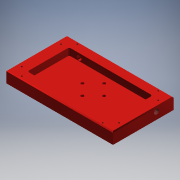
# Autodesk Inventor part: UNLHEP-14-01-P-004_ChuckForGantry
Saved by Autodesk Inventor 2019.4 (Build 234330000, 330)
## iProperties
Created: 2014-01-09
Part Number: UNLHEP-14-01-P-004_ChuckForGantry
Material: Aluminum, Anodized Red
Document SubType Name: Modeling
Designer: Frank Meier
Density: 2.7 g/cm^3
Project: UNL Pixel Phase I
Mass: 2699.72 g
Surface Area: 1115.91 cm^2
Volume: 999.896 cm^3
Appearance: Anodized - Red
Author: Frank Meier
Revision Number: 00
Autodesk Inventor part; units mm, degrees
ref_plane "YZ Plane" through (0, 0, 0) normal (1, 0, 0) x (0, 1, 0)
ref_plane "XZ Plane" through (0, 0, 0) normal (0, 1, 0) x (-1, 0, 0)
ref_plane "XY Plane" through (0, 0, 0) normal (0, 0, 1) x (1, 0, 0)
sketch "Skizze1" plane through (0, 0, 0) normal (0, 0, 1) x (1, 0, 0)
  line L0 (-123, -70) -> (123, -70)
  line L1 (123, -70) -> (123, 70)
  line L2 (123, 70) -> (-123, 70)
  line L3 (-123, 70) -> (-123, -70)
  line L4 (-123, -70) -> (123, 70) construction
  line L5 (123, -70) -> (-123, 70) construction
  point P0 (0, 0)
  dimension "d0" = 246
  dimension "d2" = 140
  constraints: 12 end point, 2 midpoint, 2 parallel, 1 horizontal, 1 perpendicular
  measures "d0" distance of L1.end L2.end
  measures "d2" distance of L0.end L1.end
extrude "Extrusion1" add sketch "Skizze1" along normal blind 26
sketch "Skizze2" plane through (0, 0, 26) normal (0, 0, 1) x (1, 0, 0)
  line L0 (-96, -48) -> (96, -48)
  line L1 (96, -48) -> (96, 48)
  line L2 (96, 48) -> (-96, 48)
  line L3 (-96, 48) -> (-96, -48)
  line L4 (-96, -48) -> (96, 48) construction
  line L5 (96, -48) -> (-96, 48) construction
  line L6 (-123, -70) -> (123, -70) projected
  line L7 (123, -70) -> (123, 70) projected
  line L8 (123, 70) -> (-123, 70) projected
  line L9 (-123, 70) -> (-123, -70) projected
  circle A0 centre (-115, 40) radius 2
  circle A1 centre (-93, 62) radius 2
  circle A2 centre (93, 62) radius 2
  circle A3 centre (115, 40) radius 2
  circle A4 centre (115, -40) radius 2
  circle A5 centre (93, -62) radius 2
  circle A6 centre (-93, -62) radius 2
  circle A7 centre (-115, -40) radius 2
  point P0 (0, 0)
  dimension "d5" = 192
  dimension "d7" = 96
  dimension "d14" = 8
  dimension "d15" = 30
  dimension "d16" = 30
  dimension "d17" = 8
  dimension "d18" = 8
  dimension "d19" = 30
  dimension "d20" = 8
  dimension "d21" = 30
  dimension "d22" = 30
  dimension "d23" = 8
  dimension "d24" = 8
  dimension "d25" = 30
  dimension "d26" = 8
  dimension "d27" = 30
  dimension "d28" = 30
  dimension "d29" = 8
  dimension "d30" = 4
  dimension "d31" = 4
  dimension "d32" = 4
  dimension "d33" = 4
  dimension "d34" = 4
  dimension "d35" = 4
  dimension "d36" = 4
  dimension "d37" = 4
  constraints: 12 end point, 8 centre point, 8 coincident, 2 midpoint, 2 parallel, 1 horizontal, 1 perpendicular
  measures "d5" distance of L1.end L2.end
  measures "d7" distance of L0.end L1.end
  measures "d14" distance from line of L9 point (-115, 40)
  measures "d15" distance from line of L8 point (-115, 40)
  measures "d16" distance from line of L9 point (-93, 62)
  measures "d17" distance from line of L8 point (-93, 62)
  measures "d18" distance from line of L8 point (93, 62)
  measures "d19" distance from line of L7 point (93, 62)
  measures "d20" distance from line of L7 point (115, 40)
  measures "d21" distance from line of L8 point (115, 40)
  measures "d22" distance from line of L6 point (115, -40)
  measures "d23" distance from line of L7 point (115, -40)
  measures "d24" distance from line of L6 point (93, -62)
  measures "d25" distance from line of L7 point (93, -62)
  measures "d26" distance from line of L6 point (-93, -62)
  measures "d27" distance from line of L9 point (-93, -62)
  measures "d28" distance from line of L6 point (-115, -40)
  measures "d29" distance from line of L9 point (-115, -40)
  measures "d30" diameter of A0
  measures "d31" diameter of A1
  measures "d32" diameter of A2
  measures "d33" diameter of A3
  measures "d34" diameter of A4
  measures "d35" diameter of A5
  measures "d36" diameter of A6
  measures "d37" diameter of A7
extrude "Extrusion2" cut sketch "Skizze2" against normal blind 16 contours L3 L2 L1 L0
fillet "Rundung1" radius 4 4 edges at (-96, 48, 18) (96, 48, 18) (96, -48, 18) (-96, -48, 18)
chamfer "Fase1" distance 2 angle 45 4 edges at (0, -70, 26) (-123, 0, 26) (0, 70, 26) (123, 0, 26)
sketch "Skizze4" plane through (0, 0, 26) normal (0, 0, 1) x (1, 0, 0)
  line L0 (123, 70) -> (-123, 70) projected
  line L1 (123, -70) -> (123, 70) projected
  line L2 (-123, 70) -> (-123, -70) projected
  line L3 (-123, -70) -> (123, -70) projected
  point P0 (-112, 45)
  point P1 (-112, -45)
  point P2 (-93, -64)
  point P3 (-93, 64)
  point P4 (93, 64)
  point P5 (112, 45)
  point P6 (112, -45)
  point P7 (93, -64)
  dimension "d153" = 25
  dimension "d154" = 25
  dimension "d155" = 11
  dimension "d156" = 6
  dimension "d157" = 30
  dimension "d158" = 11
  dimension "d159" = 6
  dimension "d160" = 30
  dimension "d161" = 30
  dimension "d162" = 6
  dimension "d163" = 11
  dimension "d164" = 25
  dimension "d165" = 11
  dimension "d166" = 25
  dimension "d167" = 6
  dimension "d168" = 30
  measures "d153" distance from line of L0 point (-112, 45)
  measures "d154" distance from line of L3 point (-112, -45)
  measures "d155" distance from line of L2 point (-112, -45)
  measures "d156" distance from line of L3 point (-93, -64)
  measures "d157" distance from line of L2 point (-93, -64)
  measures "d158" distance from line of L2 point (-112, 45)
  measures "d159" distance from line of L0 point (-93, 64)
  measures "d160" distance from line of L2 point (-93, 64)
  measures "d161" distance from line of L1 point (93, 64)
  measures "d162" distance from line of L0 point (93, 64)
  measures "d163" distance from line of L1 point (112, 45)
  measures "d164" distance from line of L0 point (112, 45)
  measures "d165" distance from line of L1 point (112, -45)
  measures "d166" distance from line of L3 point (112, -45)
  measures "d167" distance from line of L3 point (93, -64)
  measures "d168" distance from line of L1 point (93, -64)
sketch "Sketch10" plane through (123, -70, 0) normal (1, 0, 0) x (0, 0, -1)
  line L0 (-26, 138) -> (-26, 2) projected
  line L1 (0, 0) -> (-24, 0) projected
  line L2 (0, 0) -> (0, 140) projected
  point P0 (-16, 100)
  dimension "d93" = 100
  dimension "d215" = 16
  measures "d93" distance from line of L1 point (-16, 100)
  measures "d215" distance from line of L2 point (-16, 100)
hole "Bohrung3" at (123, 30, 16) direction (-1, 0, 0) diameter 10.719 depth 27 tip angle 118 taper from width 11.358 to width 10.732 over 10.02 thread size "1/4" designation "1/4 - 18 NPT" standard "NPT"
hole "Bohrung7" at (-93, 64, 26) at (-112, 45, 26) at (-112, -45, 26) at (-93, -64, 26) at (93, 64, 26) at (112, 45, 26) at (112, -45, 26) at (93, -64, 26) direction (0, 0, -1) diameter 3.242 depth 20 tip angle 118 thread size "M4x0.7" class "6H" standard "ISO Metric profile"
sketch "Sketch11" plane through (-123, 70, 0) normal (0, 1, 0) x (1, 0, 0)
  line L0 (246, 0) -> (0, 0) projected
  line L1 (0, 0) -> (0, -24) projected
  point P0 (123, 0)
  point P1 (50, -16)
  dimension "d182" = 16
  dimension "d183" = 50
  measures "d182" distance from line of L0 point (50, -16)
  measures "d183" distance from line of L1 point (50, -16)
hole "Hole8" at (-73, 70, 16) direction (0, -1, 0) diameter 10.719 depth 22 tip angle 118 taper from width 11.3588 to width 10.821 over 8.608 thread size "1/4" designation "1/4 - 18 NPT" standard "NPT for PVC Pipe and Fitting"
sketch "Sketch13" plane through (0, 0, 10) normal (0, 0, 1) x (1, 0, 0)
  circle A0 centre (-0.1124, 7.493) radius 25
  point P0 (0, 0)
  point P1 (0, 32.4927)
  point P2 (-25.1121, 7.6053)
  point P3 (-0.2247, -17.5068)
  point P4 (24.8874, 7.3806)
  dimension "d206" = 50
  dimension "d207" = 7.493
  dimension "d210" = 360
  constraints: 8 other
  measures "d207" vertical distance of point (0, 0) point (-0.112, 7.493)
hole "Hole9" at (0, 32.4927, 10) at (24.8874, 7.3806, 10) at (-0.2247, -17.5068, 10) at (-25.1121, 7.6053, 10) direction (0, 0, -1) diameter 6.6 end through all clearance for "Flat Head Machine Screw" size "M6" standard "Ansi Metric M Profile"
chamfer "Chamfer2" [suppressed]
